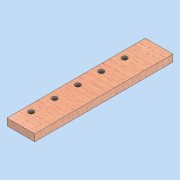
# Autodesk Inventor part: bodyBotPlate
Saved by Autodesk Inventor 2021 (Build 250183000, 183)
## iProperties
Created: 2021-02-01
Part Number: bodyBotPlate
Material: Generic
Document SubType Name: Modeling
Designer: garre
Density: 1 g/cm^3
Appearance: Default
Author: garre
Autodesk Inventor part; units mm, degrees
ref_plane "YZ Plane" through (0, 0, 0) normal (1, 0, 0) x (0, 1, 0)
ref_plane "XZ Plane" through (0, 0, 0) normal (0, 1, 0) x (-1, 0, 0)
ref_plane "XY Plane" through (0, 0, 0) normal (0, 0, 1) x (1, 0, 0)
sketch "Sketch1" plane through (0, 0, 0) normal (0, 1, 0) x (-1, 0, 0)
  line L0 (0, 0) -> (50.8, 0)
  line L1 (50.8, 0) -> (50.8, -254)
  line L2 (50.8, -254) -> (0, -254)
  line L3 (0, -254) -> (0, 0)
  dimension "d0" = 254
  dimension "d1" = 50.8
  constraints: 8 end point, 2 parallel, 1 horizontal, 1 perpendicular
  measures "d0" distance of L0.end L1.end
  measures "d1" distance of L0.start L0.end
extrude "Extrusion1" add sketch "Sketch1" along normal blind 12.7
sketch "Sketch2" plane through (0, 12.7, 0) normal (0, 1, 0) x (1, 0, 0)
  line L0 (-50.8, 0) -> (0, 0) projected
  line L1 (-38.1, 0) -> (-38.1, 850.9)
  line L2 (0, 0) -> (0, 254) projected
  line L3 (-50.8, 254) -> (-50.8, 0) projected
  circle A0 centre (-38.1, 31.75) radius 4.7625
  circle A1 centre (-38.1, 74.6125) radius 4.7625
  circle A2 centre (-38.1, 117.475) radius 4.7625
  circle A3 centre (-38.1, 160.3375) radius 4.7625
  circle A4 centre (-38.1, 203.2) radius 4.7625
  dimension "d4" = 12.7
  dimension "d5" = 31.75
  dimension "d6" = 9.525
  dimension "d7" = 42.8625
  dimension "d8" = 42.8625
  dimension "d9" = 42.8625
  dimension "d10" = 42.8625
  constraints: 6 point on line, 5 centre point, 4 equal radius, 2 end point, 1 parallel
  measures "d4" distance between parallel lines of L3 L1
  measures "d5" distance from line of L0 A0.centre
  measures "d6" diameter of A0
  measures "d7" distance of A1.centre A0.centre
  measures "d8" distance of A2.centre A1.centre
  measures "d9" distance of A3.centre A2.centre
  measures "d10" distance of A4.centre A3.centre
extrude "Extrusion2" cut sketch "Sketch2" against normal up to surface (12.7 mm away)
equation "\"d0\" = botPlateLength"
equation "\"d1\" = botPlateWidth"
equation "\"d2\" = woodThickness"
equation "\"d4\" = tuningPegOffset"
equation "\"d5\" = tuningPegEndOffset"
equation "\"d6\" = tuningPegDiameter"
equation "\"d7\" = tuningPegSeparation"
equation "\"d8\" = tuningPegSeparation"
equation "\"d9\" = tuningPegSeparation"
equation "\"d10\" = tuningPegSeparation"
equation "\"botPlateWidth\" = 50.8"
equation "\"woodThickness\" = 12.7"
equation "\"stringLength\" = 647.7"
equation "\"neckLength\" = 203.2"
equation "\"tuningPegOffset\" = 12.7"
equation "\"tuningPegDiameter\" = 9.525"
equation "\"tuningPegEndOffset\" = 31.75"
equation "\"botPlateLength\" = 254"
equation "\"tuningPegSeparation\" = 42.8625"
body "Solid1"
